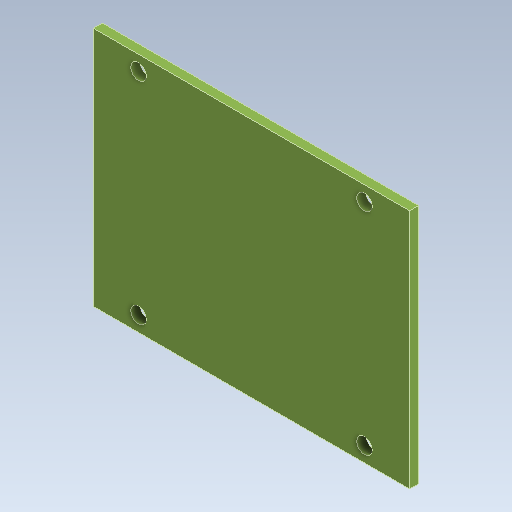
# Autodesk Inventor part: Mechanical Driver Board
Saved by Autodesk Inventor 2021 (Build 250183000, 183)
## iProperties
Created: 2019-11-04
Part Number: Mechanical Driver Board
Material: Generic
Document SubType Name: Modeling
Designer: jgray
Density: 1 g/cm^3
Appearance: Default
Author: jgray
Autodesk Inventor part; units mm, degrees
ref_plane "YZ Plane" through (0, 0, 0) normal (1, 0, 0) x (0, 1, 0)
ref_plane "XZ Plane" through (0, 0, 0) normal (0, 1, 0) x (-1, 0, 0)
ref_plane "XY Plane" through (0, 0, 0) normal (0, 0, 1) x (1, 0, 0)
sketch "Sketch1" plane through (0, 0, 0) normal (0, 0, 1) x (1, 0, 0)
  line L0 (0, 0) -> (63, 0)
  line L1 (63, 0) -> (63, 48)
  line L2 (63, 48) -> (0, 48)
  line L3 (0, 48) -> (0, 0)
  line L4 (9, 45) -> (54, 45) construction
  line L5 (54, 45) -> (54, 3) construction
  line L6 (54, 3) -> (9, 3) construction
  line L7 (9, 3) -> (9, 45) construction
  dimension "d0" = 63
  dimension "d1" = 48
  dimension "d2" = 45
  dimension "d3" = 42
  dimension "d4" = 3
  dimension "d5" = 9
  dimension "d6" = 9
  dimension "d7" = 3
  constraints: 16 end point, 4 coincident, 4 parallel, 2 horizontal, 2 perpendicular
  measures "d0" distance of L2.end L1.end
  measures "d1" distance of L1.end L0.end
  measures "d2" distance of L5.end L6.end
  measures "d3" distance of L4.end L5.end
  measures "d4" distance between parallel lines of L2 L4
  measures "d5" distance between parallel lines of L1 L5
  measures "d6" distance between parallel lines of L7 L3
  measures "d7" distance between parallel lines of L0 L6
extrude "Extrusion1" add sketch "Sketch1" along normal blind 1.8
hole "Hole1" at (9, 45, 0) at (54, 45, 0) at (9, 3, 0) at (54, 3, 0) direction (0, 0, 1) diameter 3.1 end through all
body "Solid1"
